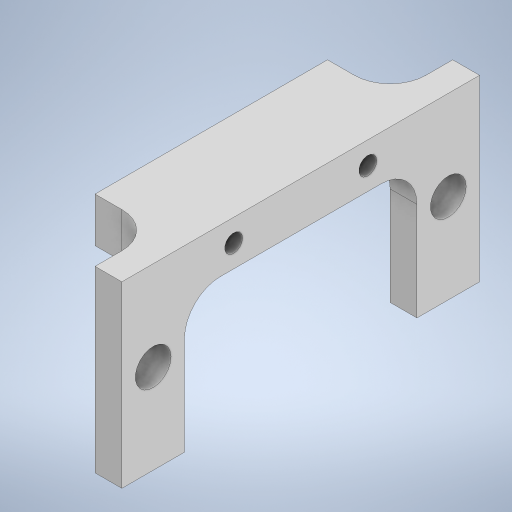
# Autodesk Inventor part: mpu6050
Saved by Autodesk Inventor 2024.2 (Build 282272000, 272)
## iProperties
Created: 2024-06-04
Part Number: mpu6050
Material: Generic
Document SubType Name: Modeling
Designer: Robin
Density: 1 g/cm^3
Appearance: Default
Author: Robin
Autodesk Inventor part; units mm, degrees
ref_plane "YZ Plane" through (0, 0, 0) normal (1, 0, 0) x (0, 1, 0)
ref_plane "XZ Plane" through (0, 0, 0) normal (0, 1, 0) x (-1, 0, 0)
ref_plane "XY Plane" through (0, 0, 0) normal (0, 0, 1) x (1, 0, 0)
sketch "Sketch1" plane through (0, 0, 0) normal (0, 1, 0) x (-1, 0, 0)
  line L0 (10, 20) -> (0, 20)
  line L1 (0, 20) -> (0, -20)
  line L2 (0, -20) -> (10, -20)
  line L3 (10, -20) -> (10, 20)
  line L4 (10, 20) -> (3, 20)
  line L5 (3, 20) -> (3, 13)
  line L6 (3, 13) -> (10, 13)
  line L7 (10, 13) -> (10, 20)
  line L8 (10, -20) -> (3, -20)
  line L9 (3, -20) -> (3, -13)
  line L10 (3, -13) -> (10, -13)
  line L11 (10, -13) -> (10, -20)
  point P0 (0, 0)
  point P1 (0, 0)
  dimension "d0" = 10
  dimension "d1" = 40
  dimension "d2" = 7
  dimension "d3" = 7
  dimension "d4" = 7
  dimension "d5" = 7
  constraints: 24 end point, 6 parallel, 3 horizontal, 3 perpendicular, 1 coincident, 1 midpoint, 1 vertical alignment
  measures "d0" distance between parallel lines of L1 L3
  measures "d1" distance of L2.end L0.start
  measures "d2" distance of L6.end L5.end
  measures "d3" distance of L5.end L4.end
  measures "d4" distance of L9.end L10.end
  measures "d5" distance of L8.end L9.end
extrude "Extrusion1" add sketch "Sketch1" along normal blind 20 contours L5 L6 L3 L10 L9 L2 L1 L0
sketch "Sketch2" plane through (-10, 0, -13) normal (-1, 0, 0) x (0, 0, 1)
  line L0 (0, 0) -> (26, 0) projected
  line L1 (0, 0) -> (0, 20) projected
  line L2 (26, 0) -> (0, 0)
  line L3 (0, 0) -> (0, 15)
  line L4 (0, 15) -> (26, 15)
  line L5 (26, 15) -> (26, 0)
  circle A0 centre (29.5, 10) radius 2
  circle A1 centre (-3.5, 10) radius 2
  line L6 (-7, 0) -> (-7, 20) projected
  line L7 (26, 0) -> (33, 0) projected
  line L8 (-7, 0) -> (0, 0) projected
  point P0 (13, 0)
  point P1 (-7, 10)
  point P2 (29.5, 0)
  point P3 (-3.5, 0)
  dimension "d8" = 15
  dimension "d9" = 4
  dimension "d10" = 4
  constraints: 8 end point, 3 midpoint, 2 centre point, 2 horizontal alignment, 2 parallel, 2 vertical alignment, 1 horizontal, 1 perpendicular, 1 point on line
  measures "d8" distance between parallel lines of L0 L4
  measures "d9" diameter of A0
  measures "d10" diameter of A1
extrude "Extrusion2" cut sketch "Sketch2" against normal through all
sketch "Sketch3" plane through (-10, 20, -13) normal (-1, 0, 0) x (0, 0, 1)
  circle A0 centre (20.5, -2.5) radius 1
  circle A1 centre (5.5, -2.5) radius 1
  line L0 (0, -5) -> (0, 0) projected
  line L1 (20.5, -2.5) -> (5.5, -2.5)
  line L2 (0, -5) -> (26, -5) projected
  point P0 (13, -20)
  point P1 (0, -2.5)
  point P2 (13, -2.5)
  point P3 (13, -5)
  dimension "d13" = 2
  dimension "d14" = 2
  dimension "d15" = 15
  constraints: 3 midpoint, 2 centre point, 2 end point, 2 horizontal alignment, 1 horizontal, 1 vertical alignment
  measures "d13" diameter of A0
  measures "d14" diameter of A1
  measures "d15" distance of L1.start L1.end
extrude "Extrusion3" cut sketch "Sketch3" against normal through all
fillet "Fillet1" radius 4 4 edges at (-3, 17.5, -13) (-3, 17.5, 13) (-1.5, 15, -13) (-1.5, 15, 13)
fillet "Fillet2" radius 2 4 edges at (-3, 15, 15) (-3, 15, 11) (-3, 15, -15) (-3, 15, -11)
body "Solid1"
